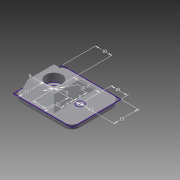
# Autodesk Inventor part: keithley_2000_rear_feet
Saved by Autodesk Inventor 2015 (Build 190159000, 159)
## iProperties
Created: 2015-05-21
Part Number: keithley_2000_rear_feet
Material: Generic
Document SubType Name: Modeling
Designer: Justin
Density: 1 g/cm^3
Appearance: Default
Author: Justin
Autodesk Inventor part; units mm, degrees
ref_plane "YZ Plane" through (0, 0, 0) normal (1, 0, 0) x (0, 1, 0)
ref_plane "XZ Plane" through (0, 0, 0) normal (0, 1, 0) x (-1, 0, 0)
ref_plane "XY Plane" through (0, 0, 0) normal (0, 0, 1) x (1, 0, 0)
sketch "Sketch1" plane through (0, 0, 0) normal (0, 0, 1) x (1, 0, 0)
  line L0 (0, 0) -> (36, 0)
  line L1 (36, 0) -> (36, 30)
  line L2 (36, 30) -> (0, 30)
  line L3 (0, 30) -> (0, 0)
  circle A0 centre (10, 15) radius 2.5
  circle A1 centre (26, 15) radius 2.25
  line L4 (0, 0) -> (36, 0)
  line L5 (2, 7) -> (18, 7)
  line L6 (18, 7) -> (18, 23)
  line L7 (18, 23) -> (2, 23)
  line L8 (2, 23) -> (2, 7)
  circle A2 centre (10, 15) radius 5
  dimension "d0" = 10
  dimension "d1" = 16
  dimension "d2" = 4.5
  dimension "d3" = 5
  dimension "d4" = 15
  dimension "d5" = 15
  dimension "d6" = 10
  dimension "d7" = 15
  dimension "d15" = 10
  dimension "d16" = 8
  dimension "d17" = 8
  dimension "d18" = 8
  dimension "d19" = 8
  constraints: 18 end point, 4 parallel, 3 centre point, 3 horizontal, 2 perpendicular, 1 coincident
  measures "d0" distance from line of L3 A0.centre
  measures "d1" distance of A1.centre A0.centre
  measures "d2" diameter of A1
  measures "d3" diameter of A0
  measures "d4" distance from line of L0 A1.centre
  measures "d5" distance from line of L0 A0.centre
  measures "d6" distance from line of L1 A1.centre
  measures "d7" distance from line of L2 A0.centre
  measures "d15" diameter of A2
  measures "d16" distance from line of A0.centre L5
  measures "d17" distance from line of L7 A2.centre
  measures "d18" distance from line of A2.centre L6
  measures "d19" distance from line of L8 A0.centre
extrude "Extrusion1" add sketch "Sketch1" against normal blind 2.5 contours L3 L2 L1 L0 | L8 L7 L6 L5 | A2
extrude "Extrusion3" add sketch "Sketch1" against normal blind 5 contours A1
extrude "Extrusion4" add sketch "Sketch1" along normal blind 5 contours L8 L7 L6 L5
chamfer "Chamfer1" distance 5 angle 45 1 edges at (18, 15, 0)
chamfer "Chamfer2" distance 5 angle 45 1 edges at (10, 7, 0)
chamfer "Chamfer4" distance 5 angle 45 1 edges at (10, 23, 0)
fillet "Fillet1" radius 5 1 edges at (36, 30, -1.25)
fillet "Fillet2" radius 5 1 edges at (0, 30, -1.25)
fillet "Fillet3" radius 5 1 edges at (36, 0, -1.25)
fillet "Fillet4" radius 5 1 edges at (0, 0, -1.25)
body "Solid1"
